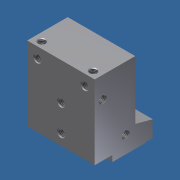
# Autodesk Inventor part: MOTOR
Saved by Autodesk Inventor 2012 SP1 (Build 160190100, 190)
## iProperties
Created: 2012-07-23
Part Number: MOTOR
Material: Default
Document SubType Name: Modeling
Designer: bruno.silveira
Density: 1 g/cm^3
Author: bruno.silveira
Autodesk Inventor part; units mm, degrees
ref_plane "YZ Plane" through (0, 0, 0) normal (1, 0, 0) x (0, 1, 0)
ref_plane "XZ Plane" through (0, 0, 0) normal (0, 1, 0) x (-1, 0, 0)
ref_plane "XY Plane" through (0, 0, 0) normal (0, 0, 1) x (1, 0, 0)
sketch "Sketch1" plane through (0, 0, 0) normal (0, 0, 1) x (1, 0, 0)
  line L0 (0, 0) -> (50, 0)
  line L1 (50, 0) -> (50, 43)
  line L2 (50, 43) -> (0, 43)
  line L3 (0, 43) -> (0, 0)
  dimension "d0" = 50
  dimension "d1" = 43
  constraints: 8 end point, 2 parallel, 1 horizontal, 1 perpendicular
  measures "d0" distance of L0.start L0.end
  measures "d1" distance of L2.end L0.start
extrude "Extrusion1" add sketch "Sketch1" along normal blind 60
sketch "Sketch2" plane through (0, 0, 0) normal (-1, 0, 0) x (0, 0, 1)
  line L0 (60, 0) -> (60, 43) projected
  line L1 (0, 43) -> (60, 43) projected
  line L2 (0, 43) -> (0, 0) projected
  line L3 (0, 0) -> (60, 0) projected
  line L4 (0, 13) -> (5, 13)
  line L5 (5, 13) -> (5, 0)
  line L6 (5, 0) -> (0, 0)
  line L7 (0, 0) -> (0, 13)
  line L8 (0, 43) -> (1, 43)
  line L9 (1, 43) -> (1, 38)
  line L10 (1, 38) -> (0, 38)
  line L11 (0, 38) -> (0, 43)
  line L12 (13, 43) -> (16.4833, 30)
  line L13 (16.4833, 30) -> (60, 30)
  dimension "d4" = 15
  dimension "d5" = 30
  dimension "d6" = 1
  dimension "d7" = 25
  dimension "d8" = 13
  dimension "d9" = 5
  constraints: 20 end point, 4 parallel, 4 point on line, 3 perpendicular, 2 horizontal
  measures "d4" angle of L2 L12
  measures "d5" distance between parallel lines of L3 L13
  measures "d6" distance between parallel lines of L2 L9
  measures "d7" distance between parallel lines of L4 L10
  measures "d8" distance of L4.end L5.end
  measures "d9" distance of L5.end L6.end
extrude "Extrusion2" cut sketch "Sketch2" against normal blind 50 contours L13 L12 L1 L0 | L3 L2 L4 L5 | L9 L10 L2 L1
sketch "Sketch3" plane through (0, 0, 60) normal (0, -1, 0) x (1, 0, 0)
  line L0 (50, -55) -> (50, 0) projected
  line L1 (50, 0) -> (0, 0) projected
  line L2 (0, -55) -> (0, 0) projected
  point P0 (0, -60)
  point P1 (7.5, -8)
  point P2 (42.5, -8)
  point P3 (25, -27.5)
  point P4 (25, -47)
  dimension "d12" = 35
  dimension "d13" = 7.5
  dimension "d14" = 27.5
  dimension "d15" = 8
  dimension "d17" = 25
  dimension "d18" = 25
  dimension "d19" = 39
  dimension "d20" = 8
  measures "d12" distance of point (42.5, -8) point (7.5, -8)
  measures "d13" distance from line of L2 point (7.5, -8)
  measures "d14" distance from line of L1 point (25, -27.5)
  measures "d15" distance from line of L1 point (7.5, -8)
  measures "d17" distance from line of L0 point (25, -47)
  measures "d18" distance from line of L0 point (25, -27.5)
  measures "d19" vertical distance of point (42.5, -8) point (25, -47)
  measures "d20" distance from line of L1 point (42.5, -8)
hole "Hole1" at (7.5, 0, 52) at (42.5, 0, 52) at (25, 0, 32.5) at (25, 0, 13) direction (0, 1, 0) diameter 4.917 depth 8 tip angle 118 thread size "M6x1" class "6H" standard "ANSI Metric M Profile"
chamfer "Chamfer1" distance 0.5 angle 45 4 edges at (7.5, 0, 54.4585) (42.5, 0, 54.4585) (25, 0, 34.9585) (25, 0, 15.4585)
sketch "Sketch4" plane through (0, 13, 0) normal (-1, 0, 0) x (0, 0, 1)
  line L0 (5, -13) -> (60, -13) projected
  line L1 (60, -13) -> (60, 17) projected
  point P0 (0, -13)
  point P1 (13, 10)
  point P2 (44, -7)
  dimension "d31" = 31
  dimension "d32" = 16
  dimension "d33" = 17
  dimension "d34" = 6
  measures "d31" horizontal distance of point (44, -7) point (13, 10)
  measures "d32" distance from line of L1 point (44, -7)
  measures "d33" vertical distance of point (13, 10) point (44, -7)
  measures "d34" distance from line of L0 point (44, -7)
hole "Hole2" at (0, 23, 13) at (0, 6, 44) direction (1, 0, 0) diameter 4.917 depth 8 tip angle 118 thread size "M6x1" class "6H" standard "ANSI Metric M Profile"
chamfer "Chamfer2" distance 0.5 angle 45 2 edges at (0, 6, 41.5415) (0, 23, 10.5415)
sketch "Sketch5" plane through (50, 13, 0) normal (1, 0, 0) x (0, 0, -1)
  circle A0 centre (-13, 10) radius 2.4585 projected
  circle A1 centre (-44, -7) radius 2.4585 projected
  point P0 (0, -13)
hole "Hole3" at (50, 6, 44) at (50, 23, 13) direction (-1, 0, 0) diameter 4.917 depth 8 tip angle 118 thread size "M6x1" class "6H" standard "ANSI Metric M Profile"
chamfer "Chamfer3" distance 0.5 angle 45 2 edges at (50, 6, 46.4585) (50, 23, 15.4585)
sketch "Sketch6" plane through (0, 0, 60) normal (0, 0, 1) x (1, 0, 0)
  line L0 (0, 0) -> (0, 30) projected
  line L1 (50, 0) -> (0, 0) projected
  point P0 (6, 5)
  point P1 (44, 5)
  dimension "d55" = 5
  dimension "d56" = 5
  dimension "d57" = 38
  dimension "d58" = 6
  measures "d55" distance from line of L1 point (44, 5)
  measures "d56" distance from line of L1 point (6, 5)
  measures "d57" distance of point (44, 5) point (6, 5)
  measures "d58" distance from line of L0 point (6, 5)
hole "Hole4" at (6, 5, 60) at (44, 5, 60) direction (0, 0, -1) diameter 4.917 depth 8 tip angle 118 thread size "M6x1" class "6H" standard "ANSI Metric M Profile"
chamfer "Chamfer4" distance 0.5 angle 45 2 edges at (6, 7.4585, 60) (44, 7.4585, 60)
sketch "Sketch7" plane through (0, 0, 5) normal (0, 0, -1) x (-1, 0, 0)
  line L0 (0, 0) -> (-50, 0) projected
  line L1 (0, 13) -> (0, 0) projected
  point P0 (-42.5, 5.5)
  point P1 (-7.5, 5.5)
  dimension "d69" = 35
  dimension "d70" = 5.5
  dimension "d71" = 7.5
  measures "d69" distance of point (-7.5, 5.5) point (-42.5, 5.5)
  measures "d70" distance from line of L0 point (-7.5, 5.5)
  measures "d71" distance from line of L1 point (-7.5, 5.5)
hole "Hole5" at (42.5, 5.5, 5) at (7.5, 5.5, 5) direction (0, 0, 1) diameter 4.917 depth 8 tip angle 118 thread size "M6x1" class "6H" standard "ANSI Metric M Profile"
chamfer "Chamfer5" distance 0.5 angle 45 2 edges at (42.5, 3.0415, 5) (7.5, 3.0415, 5)
sketch "Sketch8" plane through (0, 0, 0) normal (0, 0, -1) x (-1, 0, 0)
  line L0 (0, 38) -> (-50, 38) projected
  line L1 (-50, 13) -> (-50, 38) projected
  line L2 (-50, 13) -> (0, 13) projected
  line L3 (0, 38) -> (0, 13) projected
  line L4 (-40, 38) -> (-40, 13)
  line L5 (-10, 38) -> (-10, 13)
  point P0 (0, 0)
  dimension "d82" = 30
  dimension "d83" = 10
  constraints: 4 end point, 4 point on line, 1 parallel, 1 perpendicular
  measures "d82" distance between parallel lines of L5 L4
  measures "d83" distance between parallel lines of L1 L4
extrude "Extrusion3" cut sketch "Sketch8" against normal blind 0.5 contours L3 L2 L5 L0 | L4 L2 L1 L0
sketch "Sketch9" plane through (0, 13, 5) normal (0, -1, 0) x (1, 0, 0)
  line L0 (40, -5) -> (40, -4.5) projected
  line L1 (40, -5) -> (10, -5) projected
  line L2 (38.2335, -5) -> (38, -4.4993)
  line L3 (38, -4.4993) -> (37.7665, -5)
  line L4 (38.2335, -5) -> (37.7665, -5)
  line L5 (38, -4.4993) -> (38, -5)
  point P0 (0, -5)
  dimension "d87" = 50
  dimension "d90" = 0.467
  dimension "d91" = 2
  constraints: 8 end point, 2 point on line, 1 collinear, 1 midpoint
  measures "d87" angle of L2 L3
  measures "d90" distance of L3.end L2.start
  measures "d91" distance between parallel lines of L0 L5
extrude "Extrusion4" cut sketch "Sketch9" against normal blind 25
fillet "Fillet1" radius 0.03 1 edges at (38, 25.5, 0.5007)
pattern_linear "Rectangular Pattern1" count 14 spacing 2 along (-1, 0, 0) of "Extrusion4", "Fillet1"
chamfer "Chamfer6" distance 0.5 angle 45 2 edges at (40, 25.5, 0) (10, 25.5, 0)
body "Solid1"
